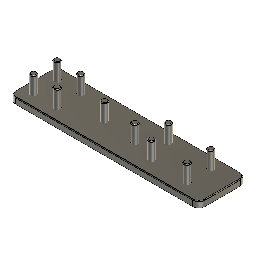
SHAPESpuzzle (Autodesk Fusion 360 design; units mm, degrees)
Autodesk Fusion 360 part; units mm, degrees
sketch "baseboard" plane through (0, 0, 0) normal (0, 0, 1) x (1, 0, 0) in component "base"
  line L0 (160, 40) -> (-160, 40)
  line L1 (-160, 40) -> (-160, -40)
  line L2 (-160, -40) -> (160, -40)
  line L3 (160, -40) -> (160, 40)
  line L4 (160, 40) -> (-160, -40) construction
  line L5 (-160, 40) -> (160, -40) construction
  line L6 (80, 40) -> (-80, 40) construction
  line L7 (-80, 40) -> (-80, -40) construction
  line L8 (-80, -40) -> (80, -40) construction
  line L9 (80, -40) -> (80, 40) construction
  line L10 (80, 40) -> (-80, -40) construction
  line L11 (-80, 40) -> (80, -40) construction
  line L12 (0, 40) -> (0, -40) construction
  line L13 (80, 40) -> (160, -40) construction
  line L14 (160, 40) -> (80, -40) construction
  line L15 (80, -40) -> (0, 40) construction
  line L16 (0, 40) -> (-80, -40) construction
  line L17 (-80, -40) -> (-160, 40) construction
  line L18 (-160, -40) -> (-80, 40) construction
  line L19 (-80, 40) -> (0, -40) construction
  line L20 (0, -40) -> (80, 40) construction
  circle A0 centre (-40, 0) radius 5
  line L21 (120, 40) -> (120, -40)
  circle A1 centre (120, 20) radius 5
  circle A2 centre (120, -20) radius 5
  circle A3 centre (56.3299, -16.3299) radius 5
  circle A4 centre (45.9772, 22.3071) radius 5
  circle A5 centre (17.6929, -5.9772) radius 5
  circle A6 centre (-100, -20) radius 5
  circle A7 centre (-100, 20) radius 5
  circle A8 centre (-140, 20) radius 5
  circle A9 centre (-140, -20) radius 5
  point P0 (120, 0)
  point P1 (-120, 0)
  point P2 (40, 0)
  dimension "d1" = 320
  dimension "d2" = 80
  dimension "d3" = 160
  dimension "d4" = 80
  dimension "d7" = 10
  dimension "d8" = 40
  dimension "d9" = 10
  dimension "d11" = 20
  dimension "d13" = 360
  dimension "d21" = 23.094
  dimension "d23" = 360
  dimension "d26" = 10
  dimension "d27" = 28.2843
  dimension "d29" = 360
  constraint horizontal L0
  constraint perpendicular L0 L1
  constraint parallel L0 L2
  constraint parallel L1 L3
  constraint coincident L4 origin
  constraint coincident L5 origin
  constraint horizontal L6
  constraint perpendicular L6 L7
  constraint parallel L6 L8
  constraint parallel L7 L9
  constraint coincident L10 origin
  constraint coincident L11 origin
  constraint midpoint L0 L12.start
  constraint midpoint L2 L12.end
  constraint midpoint L19 A0.centre
  constraint coincident L0 L21.start
  constraint coincident L2 L21.end
  constraint perpendicular L2 L21
  constraint coincident L21 A1.centre
  constraint midpoint L13 P0
  constraint midpoint L17 P1
  constraint coincident L15 A3.centre
  constraint midpoint L15 P2
  constraint coincident L17 A6.centre
  measures "d1" distance of L1.end L2.end
  measures "d2" distance of L0.end L1.end
  measures "d3" distance of L7.end L8.end
  measures "d4" distance of L6.end L7.end
  measures "d7" diameter of A0
  measures "d8" distance of L6.start L21.start
  measures "d9" diameter of A1
  measures "d11" distance of A1.centre P0
  measures "d21" distance of A3.centre P2
  measures "d26" diameter of A6
  measures "d27" distance of P1 A6.centre
extrude "Extrude1" add sketch "baseboard" along normal blind 10 contours L0 L2 L3 L21 A1 A2 | L0 L1 L2 L21 A1 A2 makes body 1 in component "base"
fillet "Fillet1" radius 10 4 edges at (-160, 40, 5) (-160, -40, 5) (160, -40, 5) (160, 40, 5) on bodies 1 in component "base"
ref_plane "WorkPlane2" through (0, 0, -40) normal (0, 0, 1) x (1, 0, 0) in component "base"
sketch "laser cutting" plane through (0, 0, -40) normal (0, 0, 1) x (1, 0, 0) in component "base"
  arc A0 (160, 30) -> (150, 40) centre (150, 30) ccw
  line L0 (150, 40) -> (-150, 40)
  arc A1 (-150, 40) -> (-160, 30) centre (-150, 30) ccw
  line L1 (-160, 30) -> (-160, -30)
  arc A2 (-160, -30) -> (-150, -40) centre (-150, -30) ccw
  line L2 (-150, -40) -> (150, -40)
  arc A3 (150, -40) -> (160, -30) centre (150, -30) ccw
  line L3 (160, -30) -> (160, 30)
  circle A4 centre (-100, 20) radius 5
  circle A5 centre (-40, 0) radius 5
  circle A6 centre (-140, 20) radius 5
  circle A7 centre (120, -20) radius 5
  circle A8 centre (56.3299, -16.3299) radius 5
  circle A9 centre (120, 20) radius 5
  circle A10 centre (-100, -20) radius 5
  circle A11 centre (17.6929, -5.9772) radius 5
  circle A12 centre (45.9772, 22.3071) radius 5
  circle A13 centre (-140, -20) radius 5
chamfer "Chamfer2" distance 1 angle 45 8 edges at (160, 0, 10) (157.0711, 37.0711, 10) (0, 40, 10) (-157.0711, 37.0711, 10) (-160, 0, 10) (-157.0711, -37.0711, 10) (0, -40, 10) (157.0711, -37.0711, 10) on bodies 1 in component "base"
extrude "Extrude1'" add sketch "baseboard" along normal blind 40 separate body contours L21 A1 | L21 A1 | L21 A2 | L21 A2 | A0 | A3 | A4 | A5 | A6 | A7 | A8 | A9 makes body 2 at (-95.0062, 19.7508, 26.6667) makes body 3 at (61.3237, -16.5792, 26.6667) makes body 4 at (-35.0062, -0.2492, 26.6667) makes body 5 at (-95.0062, -20.2492, 26.6667) makes body 6 at (124.9752, -19.5022, 26.6667) makes body 7 at (-135.0062, 19.7508, 26.6667) makes body 8 at (50.971, 22.0579, 26.6667) makes body 9 at (22.6867, -6.2264, 26.6667) makes body 10 at (-135.0062, -20.2492, 26.6667) makes body 11 at (124.9752, 20.4978, 26.6667) in component "pins"
chamfer "Chamfer1" distance 1 angle 45 10 edges at (115.3384, 18.1919, 40) (13.0313, -7.7852, 40) (-104.6616, 18.1919, 40) (-44.6616, -1.8081, 40) (41.3155, 20.499, 40) (-144.6616, 18.1919, 40) (51.6683, -18.138, 40) (-144.6616, -21.8081, 40) (115.3384, -21.8081, 40) (-104.6616, -21.8081, 40) on bodies 2 3 4 5 6 7 8 9 10 11 in component "pins"
component "base" placed x (1, 0, 0) y (0, 1, 0) z (0, 0, 1) at (0, 0, 0)
component "pins" placed x (1, 0, 0) y (0, 1, 0) z (0, 0, 1) at (0, 0, 0)
equation "d1 = unitSize * 4"
equation "d2 = unitSize"
equation "d3 = unitSize * 2"
equation "d4 = unitSize"
equation "unitSize = 80 mm"
equation "pinThickness = 10 mm"
equation "d7 = pinThickness"
equation "d8 = unitSize / 2"
equation "d9 = pinThickness"
equation "pinDistance = 40 mm"
equation "d11 = pinDistance / 2"
equation "d21 = tan(30 deg) * pinDistance"
equation "d26 = pinThickness"
equation "d27 = sqrt(2) * pinDistance / 2"
equation "roundingBase = 10 mm"
equation "chamferBase = 1 mm"
equation "roundingTile = 10 mm"
equation "chamferTile = 2 mm"
equation "d35 = roundingBase"
equation "d39 = chamferBase"
